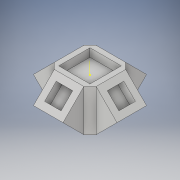
# Autodesk Inventor part: frame_nexus
Saved by Autodesk Inventor 2017 (Build 210142000, 142)
## iProperties
Created: 2017-01-19
Part Number: frame_nexus
Material: Generic
Document SubType Name: Modeling
Designer: Gabe Madonna
Density: 1 g/cm^3
Appearance: Default
Mass: 36.7878 g
Surface Area: 96.3592 cm^2
Volume: 36.7878 cm^3
Author: Gabe Madonna
Autodesk Inventor part; units mm, degrees
ref_plane "YZ Plane" through (0, 0, 0) normal (1, 0, 0) x (0, 1, 0)
ref_plane "XZ Plane" through (0, 0, 0) normal (0, 1, 0) x (-1, 0, 0)
ref_plane "XY Plane" through (0, 0, 0) normal (0, 0, 1) x (1, 0, 0)
sketch "Sketch1" plane through (0, 0, 0) normal (0, 1, 0) x (-1, 0, 0)
  point P0 (0, 0)
sketch "Sketch2" plane through (0, 0, 0) normal (0, 1, 0) x (-1, 0, 0)
  line L0 (9.525, -9.525) -> (-9.525, -9.525)
  line L1 (-9.525, -9.525) -> (-9.525, 9.525)
  line L2 (-9.525, 9.525) -> (9.525, 9.525)
  line L3 (9.525, 9.525) -> (9.525, -9.525)
  line L4 (-12.7, -12.7) -> (12.7, -12.7)
  line L5 (12.7, -12.7) -> (12.7, 12.7)
  line L6 (12.7, 12.7) -> (-12.7, 12.7)
  line L7 (-12.7, 12.7) -> (-12.7, -12.7)
  point P0 (0, 0)
  point P1 (0, 0)
  dimension "d0" = 19.05
  dimension "d1" = 3.175
  constraints: 16 end point, 1 coincident, 12 other
  measures "d0" distance of L2.end L0.start
  measures "d1" distance between parallel lines of L0 L4
extrude "Extrusion1" add sketch "Sketch2" along normal blind 5
sketch "Sketch3" plane through (0, 0, 0) normal (0, -1, 0) x (1, 0, 0)
  line L0 (12.7, -12.7) -> (-12.7, -12.7) projected
  line L1 (12.7, 12.7) -> (12.7, -12.7) projected
  line L2 (-12.7, 12.7) -> (12.7, 12.7) projected
  line L3 (-12.7, -12.7) -> (-12.7, 12.7) projected
  point P0 (0, 0)
extrude "Extrusion2" add sketch "Sketch3" along normal blind 20.4
sketch "Sketch4" plane through (12.7, 5, -12.7) normal (0, 0, -1) x (-1, 0, 0)
  line L0 (25.4, 0) -> (57.15, -31.75)
  line L1 (25.4, 0) -> (70.3013, 0) construction
  line L2 (25.4, -25.4) -> (25.4, 0) projected
  line L3 (25.4, -25.4) -> (50.8, -25.4)
  point P0 (12.7, -5)
  dimension "d6" = 45
  constraints: 6 end point, 2 horizontal, 1 equal length, 1 point on line
  measures "d6" angle of L0 L1
extrude "Extrusion3" add sketch "Sketch4" against normal up to surface (25.4 mm away)
pattern_circular "Circular Pattern2" count 4 over 360 about axis through (0, -10, 0) along (0, 1, 0) of "Extrusion3"
sketch "Sketch7" plane through (-12.7, -20.4, -12.7) normal (0, 0, -1) x (-1, 0, 0)
  line L0 (0, 0) -> (25.4, 0) projected
  line L1 (25.4, 0) -> (0, 25.4) projected
  line L2 (0, 0) -> (12.7, 12.7)
  point P0 (-12.7, 20.4)
  constraints: 2 end point, 1 midpoint
extrude "Extrusion6" cut sketch "Sketch7" against normal through all
sketch "Sketch8" plane through (-12.7, 5, -12.7) normal (-0.7071068, 0.7071068, 0) x (-0.7071068, -0.7071068, 0)
  line L0 (0, 0) -> (0, 25.4) projected
  line L1 (0, 12.7) -> (17.9605, 12.7)
  line L2 (17.9605, 25.4) -> (17.9605, 0) projected
  line L3 (3.9803, 17.7) -> (13.9803, 17.7)
  line L4 (13.9803, 17.7) -> (13.9803, 7.7)
  line L5 (13.9803, 7.7) -> (3.9803, 7.7)
  line L6 (3.9803, 7.7) -> (3.9803, 17.7)
  point P0 (-5.4447, 12.7)
  point P1 (8.9803, 12.7)
  point P2 (3.9803, 12.7)
  dimension "d24" = 10
  constraints: 10 end point, 4 midpoint, 1 point on line, 9 other
  measures "d24" distance of L3.start L3.end
extrude "Extrusion7" cut sketch "Sketch8" against normal blind 5
sketch "Sketch9" plane through (-12.7, 5, -12.7) normal (-0.7071068, 0.7071068, 0) x (-0.7071068, -0.7071068, 0)
  line L0 (17.9605, 0) -> (17.9605, 25.4) projected
  line L1 (17.9605, 25.4) -> (0, 25.4) projected
  line L2 (0, 0) -> (0, 25.4) projected
  line L3 (17.9605, 0) -> (0, 0) projected
  line L4 (0, 21.6803) -> (17.9605, 21.6803)
  line L5 (17.9605, 21.6803) -> (17.9605, 3.7197)
  line L6 (17.9605, 3.7197) -> (0, 3.7197)
  line L7 (0, 3.7197) -> (0, 21.6803)
  point P0 (-5.4447, 12.7)
  point P1 (8.9803, 12.7)
  point P2 (0, 12.7)
  constraints: 8 end point, 2 midpoint, 9 other
extrude "Extrusion8" cut sketch "Sketch9" against normal up to surface contours L3 L2 L6 L0 | L4 L2 L1 L0 surface through (-12.7, -7.7, -25.4) normal (-1, 0, 0)
pattern_circular "Circular Pattern3" count 4 over 360 about axis through (0, -10, 0) along (0, 1, 0) of "Extrusion8", "Extrusion6", "Extrusion7"
sketch "Sketch10" plane through (0, 5, 0) normal (0, 1, 0) x (1, 0, 0)
  line L0 (8.9803, -12.7) -> (12.7, -12.7) projected
  line L1 (12.7, -12.7) -> (12.7, -8.9803) projected
  line L2 (12.7, -8.9803) -> (8.9803, -12.7)
  point P0 (0, 0)
  constraints: 2 end point
extrude "Extrusion9" cut sketch "Sketch10" against normal through all
pattern_circular "Circular Pattern4" count 4 over 360 about axis through (0, -10, 0) along (0, 1, 0) of "Extrusion9"
body "Solid1"
